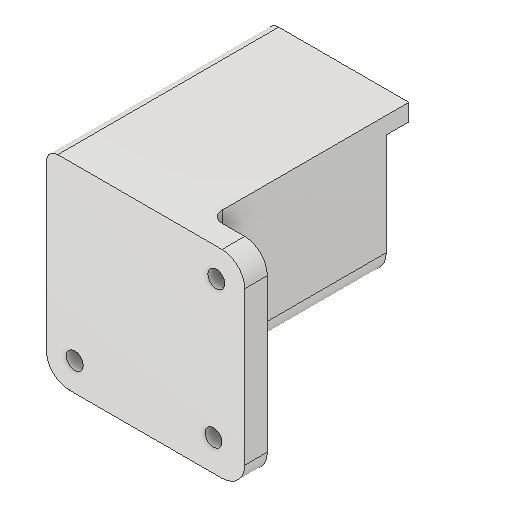
# Autodesk Inventor part: 3DP_PLA_Sorting_line_base_plate_standoff
Saved by Autodesk Inventor 2025 (Build 290162010, 162A)
## iProperties
Created: 2018-08-02
Part Number: 3DP_PLA_Sorting_line_base_plate_standoff
Material: ABS Plastic
Document SubType Name: Modeling
Designer: Andrzej
Density: 1.06 g/cm^3
Appearance: Smooth - White
Author: Andrzej
Autodesk Inventor part; units mm, degrees
ref_plane "YZ Plane" through (0, 0, 0) normal (1, 0, 0) x (0, 1, 0)
ref_plane "XZ Plane" through (0, 0, 0) normal (0, 1, 0) x (-1, 0, 0)
ref_plane "XY Plane" through (0, 0, 0) normal (0, 0, 1) x (1, 0, 0)
sketch "Sketch1" plane through (0, 0, 0) normal (0, 0, 1) x (1, 0, 0)
  line L0 (-12.7278, 13.5367) -> (12.2722, 13.5367)
  line L1 (12.2722, 13.5367) -> (12.2722, -11.4633)
  line L2 (12.2722, -11.4633) -> (-12.7278, -11.4633)
  line L3 (-12.7278, -11.4633) -> (-12.7278, 13.5367)
  line L4 (-9.7278, -11.4633) -> (-9.7278, 10.5367)
  line L5 (-9.7278, 10.5367) -> (12.2722, 10.5367)
  point P0 (0, 0)
  point P1 (1.2722, -0.4633)
  dimension "d0" = 25
  dimension "d1" = 25
  dimension "d2" = 3
  dimension "d3" = 3
  dimension "d4" = 11
  dimension "d5" = 11
  constraints: 12 end point, 2 parallel, 2 perpendicular, 2 point on line, 1 horizontal, 1 vertical
  measures "d0" distance of L1.end L2.end
  measures "d1" distance of L0.end L1.end
  measures "d2" distance between parallel lines of L3 L4
  measures "d3" distance between parallel lines of L0 L5
  measures "d4" distance from line of L2 point (1.272, -0.463)
  measures "d5" distance from line of L1 point (1.272, -0.463)
extrude "Extrusion1" add sketch "Sketch1" along normal blind 35
extrude "Extrusion2" add sketch "Sketch1" against normal blind 4 contours L0 L1 L5 L4 L2 L3
hole "Hole1" at (1.2722, -0.4633, 0) direction (0, 0, 1) diameter 4.5 depth 15 tip angle 118
sketch "Sketch2" plane through (0, 0, 35) normal (0, 0, 1) x (1, 0, 0)
  line L0 (-12.7278, 13.5367) -> (-12.7278, -11.4633) projected
  line L1 (-12.7278, -11.4633) -> (12.2722, -11.4633) projected
  line L2 (12.2722, -11.4633) -> (12.2722, 13.5367) projected
  line L3 (12.2722, 13.5367) -> (-12.7278, 13.5367) projected
  line L4 (12.2722, 13.5367) -> (12.2722, 10.5367) projected
  line L5 (12.2722, 13.5367) -> (22.2722, 13.5367)
  line L6 (22.2722, 13.5367) -> (22.2722, -21.4633)
  line L7 (22.2722, -21.4633) -> (-12.7278, -21.4633)
  line L8 (-12.7278, -21.4633) -> (-12.7278, -11.4633)
  point P0 (0, 0)
  point P1 (17.2722, 8.5367)
  point P2 (-7.7278, -16.4633)
  point P3 (16.7722, -15.9633)
  dimension "d17" = 10
  dimension "d18" = 10
  dimension "d21" = 5
  dimension "d22" = 5
  dimension "d23" = 5.5
  dimension "d24" = 5.5
  dimension "d25" = 5
  dimension "d26" = 5
  constraints: 8 end point, 2 horizontal, 1 collinear, 1 perpendicular
  measures "d17" distance of L2.end L5.end
  measures "d18" distance of L7.end L0.end
  measures "d21" distance from line of L6 point (17.272, 8.537)
  measures "d22" distance from line of L7 point (-7.728, -16.463)
  measures "d23" distance from line of L6 point (16.772, -15.963)
  measures "d24" distance from line of L7 point (16.772, -15.963)
  measures "d25" distance from line of point (17.272, 8.537) L5
  measures "d26" distance from line of L8 point (-7.728, -16.463)
extrude "Extrusion3" add sketch "Sketch2" against normal blind 4 contours L1 L2 L5 L6 L7 L8
hole "Hole2" at (17.2722, 8.5367, 35) at (-7.7278, -16.4633, 35) at (16.7722, -15.9633, 35) direction (0, 0, -1) diameter 3 end through all
chamfer "Chamfer1" distance 1.5 angle 45 3 edges at (16.7722, -14.4633, 31) (17.2722, 10.0367, 31) (-7.7278, -14.9633, 31)
fillet "Fillet1" radius 4 4 edges at (22.2722, -21.4633, 33) (-12.7278, -21.4633, 33) (22.2722, 13.5367, 33) (12.2722, -11.4633, 15.5)
fillet "Fillet2" radius 2 4 edges at (-12.7278, 13.5367, 15.5) (11.1006, -10.2917, 31) (12.2722, 3.0367, 31) (-2.2278, -11.4633, 31)
equation "\"d3\" = d2"
equation "\"d22\" = d21"
equation "\"d24\" = d23"
equation "\"d26\" = d25"
body "Solid1"
